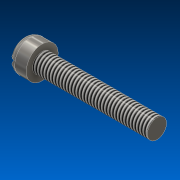
# Autodesk Inventor part: parafuso do captador( necessita de reparo)
Saved by Autodesk Inventor 2016 (Build 200138000, 138)
## iProperties
Created: 2018-12-07
Part Number: parafuso do captador( necessita de reparo)
Material: Generic
Document SubType Name: Modeling
Designer: lesly
Density: 1 g/cm^3
Appearance: Steel - Polished
Author: lesly
Autodesk Inventor part; units mm, degrees
ref_plane "YZ Plane" through (0, 0, 0) normal (1, 0, 0) x (0, 1, 0)
ref_plane "XZ Plane" through (0, 0, 0) normal (0, 1, 0) x (-1, 0, 0)
ref_plane "XY Plane" through (0, 0, 0) normal (0, 0, 1) x (1, 0, 0)
sketch "Sketch1" plane through (0, 0, 0) normal (1, 0, 0) x (0, 1, 0)
  circle A0 centre (0, 0) radius 2.5
  constraints: 1 centre point, 1 coincident
extrude "Extrusion1" add sketch "Sketch1" along normal mid plane 3
sketch "Sketch2" plane through (1.5, 0, 0) normal (1, 0, 0) x (0, 0, -1)
  circle A0 centre (0, 0) radius 1.5
  constraints: 1 centre point, 1 coincident
extrude "Extrusion2" add sketch "Sketch2" along normal blind 18
fillet "Fillet1" radius 1.2 1 edges at (-1.5, -2.5, 0)
sketch "Sketch3" plane through (0, 0, 0) normal (0, 1, 0) x (-1, 0, 0)
  line L0 (1.5, 1.3) -> (1.5, -1.3) projected
  line L1 (0.3, -2.5) -> (0.3, 2.5) projected
  line L2 (1.5, 0.5) -> (0.3, 0.5)
  line L3 (1.5, -0.5) -> (0.3, -0.5)
  line L4 (1.5, -0.5) -> (1.5, 0.5)
  line L5 (0.3, 0.5) -> (0.3, -0.5)
  point P0 (0, 0)
  constraints: 8 end point, 2 collinear
extrude "Extrusion3" cut sketch "Sketch3" along normal mid plane 18
thread "Thread1" size "M3x0.5" class "6g" standard "ANSI Metric M Profile" full length
thread "Thread2" size "M3x0.5" class "6g" standard "ANSI Metric M Profile" full length
body "Solid1"
